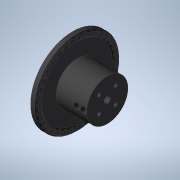
# Autodesk Inventor part: Pulley
Saved by Autodesk Inventor 2021 (Build 250183000, 183)
## iProperties
Created: 2024-01-31
Part Number: Pulley
Material: Generic
Document SubType Name: Modeling
Designer: Lukas
Density: 1 g/cm^3
Appearance: Default
Author: Lukas
Autodesk Inventor part; units mm, degrees
ref_plane "YZ Plane" through (0, 0, 0) normal (1, 0, 0) x (0, 1, 0)
ref_plane "XZ Plane" through (0, 0, 0) normal (0, 1, 0) x (-1, 0, 0)
sketch "Sketch1" plane through (0, 0, 0) normal (0, 0, 1) x (1, 0, 0)
  line L0 (0, 19) -> (26, 19)
  line L1 (26, 19) -> (26, 4)
  line L2 (26, 4) -> (42, 4)
  line L3 (42, 4) -> (42, 25)
  line L4 (42, 25) -> (5, 25)
  line L5 (5, 25) -> (5, 43)
  line L6 (5, 43) -> (7, 45)
  line L7 (7, 45) -> (7, 49)
  line L8 (7, 49) -> (5, 51)
  line L9 (5, 51) -> (0, 51)
  line L10 (0, 51) -> (0, 19)
  line L11 (-8.4, 0) -> (50.4, 0) projected
  point P0 (0, 0)
  dimension "d0" = 4
  dimension "d1" = 19
  dimension "d2" = 26
  dimension "d3" = 16
  dimension "d4" = 2
  dimension "d5" = 2
  dimension "d6" = 2
  dimension "d7" = 45
  dimension "d8" = 25
  dimension "d9" = 5
  dimension "d10" = 4
  constraints: 22 end point, 6 perpendicular, 2 parallel, 1 horizontal, 1 point on line, 1 vertical alignment
  measures "d0" distance from line of point (0, 0) L2
  measures "d1" distance from line of point (0, 0) L0
  measures "d2" distance from line of L1 point (0, 0)
  measures "d3" distance of L1.end L2.end
  measures "d4" horizontal distance of L7.end L8.end
  measures "d5" horizontal distance of L5.end L6.end
  measures "d6" distance between parallel lines of L7 L5
  measures "d7" vertical distance of L6.end point (0, 0)
  measures "d8" distance from line of L4 point (0, 0)
  measures "d9" distance between parallel lines of L10 L5
  measures "d10" distance of L6.end L7.end
revolve "Revolution1" add sketch "Sketch1" angle 360 about axis through (-10, 0, 0) along (1, 0, 0)
sketch "Sketch2" plane through (0, 0, 0) normal (0, 0, 1) x (1, 0, 0)
  circle A0 centre (30, 0) radius 1.4
  circle A1 centre (38, 0) radius 1.4
  point P0 (0, 0)
  dimension "d12" = 2.8
  dimension "d13" = 30
  dimension "d14" = 8
  constraints: 2 centre point, 2 horizontal alignment, 1 equal radius
  measures "d12" diameter of A0
  measures "d13" distance of point (0, 0) A0.centre
  measures "d14" distance of A1.centre A0.centre
extrude "Extrusion1" cut sketch "Sketch2" along normal through all
ref_plane "Work Plane1" through (0, 0, 30) normal (0, 0, 1) x (1, 0, 0)
sketch "Sketch3" plane through (0, 0, 30) normal (0, 0, 1) x (1, 0, 0)
  circle A0 centre (30, 0) radius 3.75
  circle A1 centre (38, 0) radius 3.75
  spline S0 degree 7 poles (39.4, 0) (39.4, 0.1983) (39.3672, 0.3916) (39.3047, 0.5736) (39.2166, 0.7392) (39.1083, 0.8844) (38.9863, 1.0067) (38.7481, 1.1915) (38.6312, 1.2618) (38.5093, 1.3174) (38.3841, 1.3588) (38.2568, 1.3863) (38.1284, 1.4) (37.8321, 1.4) (37.6643, 1.3765) (37.4986, 1.3295) (37.3377, 1.2585) (37.1847, 1.1625) (37.0439, 1.0406) (36.8125, 0.7609) (36.715, 0.6049) (36.639, 0.4276) (36.5919, 0.2351) (36.5774, 0.0359) (36.596, -0.1611) (36.6752, -0.4699) (36.7192, -0.5883) (36.7756, -0.7019) (36.8436, -0.809) (36.9223, -0.9084) (37.0108, -0.9986) (37.2141, -1.1668) (37.3308, -1.2427) (37.4559, -1.3048) (37.5875, -1.3522) (37.7235, -1.3841) (37.8618, -1.4) (38.1284, -1.4) (38.2568, -1.3863) (38.3841, -1.3588) (38.5093, -1.3174) (38.6312, -1.2618) (38.7481, -1.1915) (38.9863, -1.0068) (39.1083, -0.8844) (39.2166, -0.7392) (39.3047, -0.5735) (39.3673, -0.3915) (39.4, -0.1982) (39.4, 0) knots 0 0 0 0 0 0 0 0 0.14782 0.14782 0.14782 0.14782 0.14782 0.14782 0.274597 0.274597 0.274597 0.274597 0.274597 0.274597 0.440349 0.440349 0.440349 0.440349 0.440349 0.440349 0.587367 0.587367 0.587367 0.587367 0.587367 0.587367 0.683042 0.683042 0.683042 0.683042 0.683042 0.683042 0.788293 0.788293 0.788293 0.788293 0.788293 0.788293 0.886053 0.886053 0.886053 0.886053 0.886053 0.886053 1 1 1 1 1 1 1 1 projected
  spline S1 degree 7 poles (31.4, 0) (31.4, 0.1983) (31.3672, 0.3916) (31.3047, 0.5736) (31.2166, 0.7392) (31.1083, 0.8844) (30.9863, 1.0067) (30.7481, 1.1915) (30.6312, 1.2618) (30.5093, 1.3174) (30.3841, 1.3588) (30.2568, 1.3863) (30.1284, 1.4) (29.8321, 1.4) (29.6643, 1.3765) (29.4986, 1.3295) (29.3377, 1.2585) (29.1847, 1.1625) (29.0439, 1.0406) (28.8125, 0.7609) (28.715, 0.6049) (28.639, 0.4276) (28.5919, 0.2351) (28.5774, 0.0359) (28.596, -0.1611) (28.6752, -0.4699) (28.7192, -0.5883) (28.7756, -0.7019) (28.8436, -0.809) (28.9223, -0.9084) (29.0108, -0.9986) (29.2141, -1.1668) (29.3308, -1.2427) (29.4559, -1.3048) (29.5875, -1.3522) (29.7235, -1.3841) (29.8618, -1.4) (30.1284, -1.4) (30.2568, -1.3863) (30.3841, -1.3588) (30.5093, -1.3174) (30.6312, -1.2618) (30.7481, -1.1915) (30.9863, -1.0068) (31.1083, -0.8844) (31.2166, -0.7392) (31.3047, -0.5735) (31.3673, -0.3915) (31.4, -0.1982) (31.4, 0) knots 0 0 0 0 0 0 0 0 0.14782 0.14782 0.14782 0.14782 0.14782 0.14782 0.274597 0.274597 0.274597 0.274597 0.274597 0.274597 0.440349 0.440349 0.440349 0.440349 0.440349 0.440349 0.587367 0.587367 0.587367 0.587367 0.587367 0.587367 0.683042 0.683042 0.683042 0.683042 0.683042 0.683042 0.788293 0.788293 0.788293 0.788293 0.788293 0.788293 0.886053 0.886053 0.886053 0.886053 0.886053 0.886053 1 1 1 1 1 1 1 1 projected
  point P0 (0, 0)
  dimension "d18" = 7.5
  constraints: 2 centre point, 2 horizontal alignment, 2 vertical alignment, 1 equal radius, 4 other
  measures "d18" diameter of A0
extrude "Extrusion2" cut sketch "Sketch3" against normal blind 12
sketch "Sketch4" plane through (0, 0, 30) normal (0, 0, 1) x (1, 0, 0)
  line L0 (7, -49) -> (7, 49) projected
  line L1 (7, -45) -> (7, 45) projected
  line L2 (7, -2.5) -> (6, -1.5)
  line L3 (6, -1.5) -> (6, 1.5)
  line L4 (6, 1.5) -> (7, 2.5)
  point P0 (0, 0)
  point P1 (6, 0)
  point P2 (7, 0)
  dimension "d21" = 1
  dimension "d22" = 1
  dimension "d23" = 3
  dimension "d25" = 1
  constraints: 6 end point, 2 midpoint, 2 point on line, 1 horizontal alignment, 1 vertical
  measures "d21" horizontal distance of L2.start L2.end
  measures "d22" horizontal distance of L3.end L4.end
  measures "d23" distance of L2.end L3.end
  measures "d25" distance between parallel lines of L0 L3
extrude "Extrusion3" cut sketch "Sketch4" along normal through all
pattern_circular "Circular Pattern1" count 36 over 360 about axis through (-10, 0, 0) along (1, 0, 0) of "Extrusion3"
sketch "Sketch5" plane through (42, 0, 0) normal (1, 0, 0) x (0, 0, -1)
  circle A0 centre (-10, 10) radius 2.1
  circle A1 centre (10, -10) radius 2.1
  circle A2 centre (10, 10) radius 2.1
  circle A3 centre (-10, -10) radius 2.1
  circle A4 centre (-10, -10) radius 1.6
  circle A5 centre (-10, 10) radius 1.6
  circle A6 centre (10, 10) radius 1.6
  circle A7 centre (10, -10) radius 1.6
  point P0 (0, 0)
  dimension "d31" = 20
  dimension "d32" = 20
  dimension "d33" = 10
  dimension "d34" = 10
  dimension "d35" = 4.2
  dimension "d38" = 3.2
  constraints: 8 centre point, 6 equal radius, 4 coincident, 2 horizontal alignment, 2 vertical alignment
  measures "d31" distance of A2.centre A0.centre
  measures "d32" distance of A2.centre A1.centre
  measures "d33" horizontal distance of point (0, 0) A0.centre
  measures "d34" horizontal distance of point (0, 0) A2.centre
  measures "d35" diameter of A3
  measures "d38" diameter of A5
extrude "Extrusion4" cut sketch "Sketch5" against normal blind 6.2 contours A0 | A1 | A2 | A3 | A4 | A5 | A6 | A7
extrude "Extrusion5" cut sketch "Sketch5" against normal through all contours A4 | A5 | A6 | A7
equation "\"d5\" = d4"
equation "\"d22\" = d21"
equation "\"d32\" = d31"
equation "\"d33\" = 0.5 * d31"
equation "\"d34\" = 0.5 * d32"
body "Solid1"
